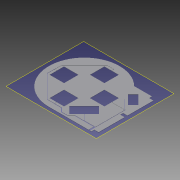
# Autodesk Inventor part: Foam_Left
Saved by Autodesk Inventor 2014 SP1 (Build 180222100, 222)
## iProperties
Created: 2014-01-12
Part Number: Foam_Left
Material: Generic
Document SubType Name: Modeling
Designer: tuleu
Density: 1 g/cm^3
Appearance: Default
Author: tuleu
Autodesk Inventor part; units mm, degrees
ref_plane "YZ Plane" through (0, 0, 0) normal (1, 0, 0) x (0, 1, 0)
ref_plane "XZ Plane" through (0, 0, 0) normal (0, 1, 0) x (-1, 0, 0)
ref_plane "XY Plane" through (0, 0, 0) normal (0, 0, 1) x (1, 0, 0)
sketch "Sketch1" plane through (0, 0, 0) normal (0, 1, 0) x (-1, 0, 0)
  line L0 (-100, 380) -> (-100, 180)
  line L1 (-100, 180) -> (100, 180)
  line L2 (100, 180) -> (100, 380)
  line L3 (-180, 100) -> (-380, 100)
  line L4 (-380, -100) -> (-180, -100)
  line L5 (-180, -100) -> (-180, 100)
  line L6 (380, 100) -> (180, 100)
  line L7 (180, 100) -> (180, -100)
  line L8 (180, -100) -> (380, -100)
  line L9 (100, -180) -> (-100, -180)
  line L10 (-100, -180) -> (-100, -380)
  line L11 (100, -380) -> (100, -180)
  line L12 (0, 380) -> (0, -380) construction
  line L13 (380, 0) -> (-380, 0) construction
  line L14 (100, 280) -> (-100, 280) construction
  line L15 (-550, 490) -> (-550, 420)
  line L16 (-570, 409) -> (-570, 490)
  line L17 (-284.2784, 420) -> (-550, 420)
  line L18 (-335.8757, 130.8148) -> (-434.8707, 229.8097)
  line L19 (-229.8097, 434.8707) -> (-130.8148, 335.8757)
  line L20 (-130.8148, 335.8757) -> (-335.8757, 130.8148)
  line L21 (-197.9899, 304.0559) -> (-304.0559, 197.9899) projected
  arc A0 (-367.6955, 261.6295) -> (-304.0559, 197.9899) centre (-335.8757, 229.8097) ccw projected
  line L22 (-367.6955, 261.6295) -> (-261.6295, 367.6955) projected
  arc A1 (-197.9899, 304.0559) -> (-261.6295, 367.6955) centre (-229.8097, 335.8757) ccw projected
  line L23 (-234.2784, 470) -> (-284.2784, 420)
  line L24 (-100, 380) -> (-100, 404.7721) construction
  line L25 (102.4853, 416) -> (1.5, 416)
  line L26 (1.5, 416) -> (1.5, 418)
  line L27 (1.5, 418) -> (-96.6863, 418)
  line L28 (-234.2784, 470) -> (-148.6863, 470)
  line L29 (-280.9646, 412) -> (-230.9646, 462)
  line L30 (-230.9646, 462) -> (-152, 462)
  line L31 (100, 410) -> (410, 100)
  line L32 (380, 100) -> (479.6874, 100) construction
  line L33 (100, 380) -> (100, 479.6874) construction
  line L34 (102.4853, 416) -> (416, 102.4853)
  line L35 (416, 102.4853) -> (416, -1.5)
  line L36 (416, -1.5) -> (413, -1.5)
  line L37 (413, -1.5) -> (413, -101.2426)
  line L38 (380, -100) -> (479.6874, -100) construction
  line L39 (100, -380) -> (100, -479.6874) construction
  line L40 (100, -410) -> (1.5, -410)
  line L41 (410, -100) -> (100, -410)
  line L42 (413, -101.2426) -> (101.2426, -413)
  line L43 (101.2426, -413) -> (-1.5, -413)
  line L44 (-1.5, -413) -> (-1.5, -380)
  line L45 (1.5, -410) -> (1.5, -380)
  line L46 (410, 1.5) -> (380, 1.5)
  line L47 (410, -1.5) -> (380, -1.5)
  line L48 (410, 100) -> (410, 1.5)
  line L49 (410, -1.5) -> (410, -100)
  line L50 (-100, -380) -> (-1.5, -380)
  line L51 (1.5, -380) -> (100, -380)
  line L52 (1.5, -380) -> (-1.5, -380) construction
  line L53 (380, -100) -> (380, -1.5)
  line L54 (380, 1.5) -> (380, 100)
  line L55 (380, 1.5) -> (380, -1.5) construction
  line L56 (-331.2795, 333.4008) -> (-409.8787, 412)
  line L57 (-333.4008, 331.2795) -> (-411.1213, 409)
  line L58 (-434.8707, 229.8097) -> (-333.4008, 331.2795)
  line L59 (-331.2795, 333.4008) -> (-229.8097, 434.8707)
  line L60 (-564, 409) -> (-411.1213, 409)
  line L61 (-409.8787, 412) -> (-280.9646, 412)
  line L62 (-1.5, 410) -> (-1.5, 380)
  line L63 (1.5, 410) -> (1.5, 380)
  line L64 (-100, 410) -> (-1.5, 410)
  line L65 (1.5, 410) -> (100, 410)
  line L66 (100, 380) -> (1.5, 380)
  line L67 (-1.5, 380) -> (-100, 380)
  line L68 (1.5, 380) -> (-1.5, 380) construction
  line L69 (-570, 409) -> (-570, -4.5)
  line L70 (-380, 1.5) -> (-564, 1.5)
  line L71 (-564, 1.5) -> (-564, 409)
  line L72 (-380, 100) -> (-380, 1.5)
  line L73 (-380, -1.5) -> (-380, -100)
  line L74 (-380, 1.5) -> (-380, -1.5) construction
  line L75 (-100, 410) -> (-152, 462)
  line L76 (-148.6863, 470) -> (-96.6863, 418)
  arc A2 (-342.9286, -350) -> (0, 490) centre (0, 0) ccw
  line L77 (-342.9286, -350) -> (-590, -350)
  line L78 (-590, 490) -> (-590, 450)
  line L79 (-590, 90) -> (-590, 50)
  line L80 (-590, -310) -> (-590, -350)
  line L81 (-550, 490) -> (0, 490)
  line L82 (-570, 490) -> (-590, 490)
  line L83 (-590, 450) -> (-650, 450)
  line L84 (-590, 90) -> (-650, 90)
  line L85 (-650, -310) -> (-650, 50)
  line L86 (-650, 90) -> (-650, 450)
  line L87 (-650, 50) -> (-590, 50)
  line L88 (-590, -310) -> (-650, -310)
  line L89 (-485.8579, -229.4975) -> (-549.4975, -165.8579) projected
  arc A3 (-514.1421, -130.5025) -> (-549.4975, -165.8579) centre (-531.8198, -148.1802) ccw projected
  line L90 (-514.1421, -130.5025) -> (-450.5025, -194.1421) projected
  arc A4 (-485.8579, -229.4975) -> (-450.5025, -194.1421) centre (-468.1802, -211.8198) ccw projected
  line L91 (-1806, 1126) -> (476, -1156)
  line L92 (-500, -180) -> (147.3272, 467.3272)
  line L93 (-401.0051, -208.2843) -> (-471.7157, -278.9949)
  line L94 (-471.7157, -278.9949) -> (-598.9949, -151.7157)
  line L95 (-598.9949, -151.7157) -> (-528.2843, -81.0051)
  line L96 (-562.3629, -4.5) -> (-444.4921, -122.3708)
  line L97 (-444.4921, -122.3708) -> (-465.7053, -143.584)
  line L98 (-463.584, -145.7053) -> (-440.2495, -122.3708)
  line L99 (-440.2495, -122.3708) -> (-561.1203, -1.5)
  line L100 (-570, -4.5) -> (-562.3629, -4.5)
  line L101 (-561.1203, -1.5) -> (-380, -1.5)
  line L102 (-528.2843, -81.0051) -> (-465.7053, -143.584)
  line L103 (-463.584, -145.7053) -> (-401.0051, -208.2843)
  line L104 (-435, 440) -> (-525, 440) projected
  dimension "d0" = 200
  dimension "d1" = 280
  dimension "d7" = 290
  dimension "d8" = 25
  dimension "d16" = 8
  dimension "d17" = 8
  dimension "d18" = 1.5
  dimension "d22" = 6
  dimension "d24" = 1.5
  dimension "d27" = 3
  dimension "d28" = 3
  dimension "d29" = 1.5
  dimension "d30" = 3
  dimension "d31" = 3
  dimension "d32" = 6
  dimension "d33" = 3
  dimension "d35" = 30
  dimension "d37" = 30
  dimension "d38" = 3
  dimension "d39" = 8
  dimension "d41" = 140
  dimension "d42" = 20
  dimension "d43" = 11
  dimension "d44" = 3
  dimension "d45" = 30
  dimension "d46" = 6
  dimension "d47" = 8
  dimension "d48" = 6
  dimension "d50" = 8
  dimension "d52" = 20
  dimension "d54" = 20
  dimension "d58" = 180
  dimension "d61" = 3
  dimension "d62" = 3
  dimension "d63" = 3
  dimension "d64" = 6
  dimension "d65" = 30
  dimension "d66" = 100
  dimension "d67" = 20
  dimension "d68" = 20
  constraints: 200 end point, 45 perpendicular, 42 parallel, 11 collinear, 10 horizontal, 8 equal length, 8 midpoint, 6 vertical, 4 point on line, 3 point on circle, 1 centre point, 25 other
  measures "d0" distance of L2.end L0.start
  measures "d1" distance between parallel lines of L13 L14
  measures "d7" distance between parallel lines of L18 L19
  measures "d8" distance between parallel lines of L21 L20
  measures "d16" distance between parallel lines of L28 L30
  measures "d17" distance between parallel lines of L23 L29
  measures "d18" distance between parallel lines of L12 L26
  measures "d22" distance between parallel lines of L31 L34
  measures "d24" distance between parallel lines of L13 L36
  measures "d27" distance between parallel lines of L41 L42
  measures "d28" distance between parallel lines of L44 L45
  measures "d29" distance between parallel lines of L12 L44
  measures "d30" distance between parallel lines of L40 L43
  measures "d31" distance between parallel lines of L47 L46
  measures "d32" distance between parallel lines of L35 L48
  measures "d33" distance between parallel lines of L37 L49
  measures "d35" distance between parallel lines of L40 L51
  measures "d37" distance between parallel lines of L54 L48
  measures "d38" distance between parallel lines of L57 L56
  measures "d39" distance between parallel lines of L17 L61
  measures "d41" distance between parallel lines of L58 L20
  measures "d42" distance between parallel lines of L59 L29
  measures "d43" distance between parallel lines of L17 L60
  measures "d44" distance between parallel lines of L62 L63
  measures "d45" distance between parallel lines of L67 L64
  measures "d46" distance between parallel lines of L65 L25
  measures "d47" distance between parallel lines of L64 L27
  measures "d48" distance between parallel lines of L69 L71
  measures "d50" distance between parallel lines of L75 L76
  measures "d52" distance between parallel lines of L78 L16
  measures "d54" distance between parallel lines of L28 L81
  measures "d58" distance between parallel lines of L95 L93
  measures "d61" distance between parallel lines of L96 L99
  measures "d62" distance between parallel lines of L97 L98
  measures "d63" distance between parallel lines of L101 L70
  measures "d64" distance between parallel lines of L100 L70
  measures "d65" distance between parallel lines of L102 L96
  measures "d66" distance between parallel lines of L94 L103
  measures "d67" distance between parallel lines of L16 L15
  measures "d68" distance between parallel lines of L17 L104
extrude "Extrusion1" add sketch "Sketch1" against normal blind 3 contours L0 L92 L3 L72 L70 L71 L60 L57 L58 L18 L20 L19 L59 L56 L61 L29 L30 L75 L64 L62 L67 | L0 L1 L2 L66 L92 L65 L31 L48 L46 L54 L6 L7 L8 L53 L47 L49 L41 L40 L45 L51 L11 L9 L10 L50 L44 L43 L42 L37 L36 L35 L34 L25 A2 L91 L93 L103 L98 L99 L73 L4 L5 L3 | L66 L63 L65 L92 | L92 L99 L101 L73 | L25 L26 L27 L76 L28 L23 L17 L15 L81 A2 L92 | A2 L77 L80 L88 L85 L91 L95 L94 L93 | L91 L85 L87 L79 L84 L86 L83 L78 L82 L16 L69 L100 L96 L97 L102 L95
ref_plane "Work Plane1" through (0, -3, 0) normal (0, -1, 0) x (1, 0, 0)
sketch "Sketch4" plane through (0, -3, 0) normal (0, -1, 0) x (1, 0, 0)
  arc A0 (0, 490) -> (342.9286, -350) centre (0, 0) ccw projected
  line L0 (550, 490) -> (0, 490) projected
  line L1 (590, 490) -> (570, 490) projected
  line L2 (590, 490) -> (590, 450) projected
  line L3 (650, 90) -> (650, 450) projected
  line L4 (650, -310) -> (650, 50) projected
  line L5 (590, 90) -> (590, 50) projected
  line L6 (342.9286, -350) -> (590, -350) projected
  line L7 (180, -100) -> (180, 100) projected
  line L8 (380, -100) -> (180, -100) projected
  line L9 (-380, 100) -> (-180, 100) projected
  line L10 (-180, 100) -> (-180, -100) projected
  line L11 (-100, -180) -> (100, -180) projected
  line L12 (-100, -380) -> (-100, -180) projected
  line L13 (-100, 180) -> (-100, 380) projected
  line L14 (100, 180) -> (-100, 180) projected
  line L15 (130.8148, 335.8757) -> (229.8097, 434.8707) projected
  line L16 (434.8707, 229.8097) -> (335.8757, 130.8148) projected
  line L17 (528.2843, -81.0051) -> (598.9949, -151.7157) projected
  line L18 (471.7157, -278.9949) -> (401.0051, -208.2843) projected
  line L19 (590, -310) -> (590, -350) projected
  line L20 (590, 450) -> (650, 450)
  line L21 (650, 450) -> (650, 90)
  line L22 (590, 90) -> (650, 90)
  line L23 (590, 90) -> (590, 50)
  line L24 (650, 50) -> (590, 50)
  line L25 (650, -310) -> (650, 50)
  line L26 (590, -310) -> (650, -310)
  line L27 (590, -310) -> (590, -350)
  line L28 (590, -350) -> (342.9286, -350)
  line L29 (0, 490) -> (590, 490)
  line L30 (590, 490) -> (590, 450)
  line L31 (229.8097, 434.8707) -> (130.8148, 335.8757)
  line L32 (130.8148, 335.8757) -> (335.8757, 130.8148)
  line L33 (335.8757, 130.8148) -> (434.8707, 229.8097)
  line L34 (434.8707, 229.8097) -> (229.8097, 434.8707)
  line L35 (528.2843, -81.0051) -> (598.9949, -151.7157)
  line L36 (598.9949, -151.7157) -> (471.7157, -278.9949)
  line L37 (471.7157, -278.9949) -> (401.0051, -208.2843)
  line L38 (401.0051, -208.2843) -> (528.2843, -81.0051)
  line L39 (-100, 380) -> (100, 380)
  line L40 (100, 380) -> (100, 180)
  line L41 (100, 180) -> (-100, 180)
  line L42 (-100, 180) -> (-100, 380)
  line L43 (-380, 100) -> (-180, 100)
  line L44 (-180, 100) -> (-180, -100)
  line L45 (-180, -100) -> (-380, -100)
  line L46 (-380, -100) -> (-380, 100)
  line L47 (180, 100) -> (380, 100)
  line L48 (380, 100) -> (380, -100)
  line L49 (380, -100) -> (180, -100)
  line L50 (180, -100) -> (180, 100)
  line L51 (100, -180) -> (-100, -180)
  line L52 (-100, -180) -> (-100, -380)
  line L53 (-100, -380) -> (100, -380)
  line L54 (100, -380) -> (100, -180)
  arc A1 (0, 490) -> (342.9286, -350) centre (0, 0) ccw
  constraints: 70 end point, 15 perpendicular, 13 parallel, 5 collinear, 4 horizontal, 2 point on circle, 1 centre point, 1 coincident, 1 tangent
extrude "Extrusion3" add sketch "Sketch4" along normal blind 3
body "Solid1"
